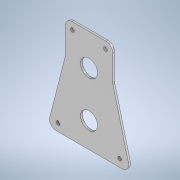
# Autodesk Inventor part: TH22_AlBoard_roller_sub_sn
Saved by Autodesk Inventor 2022 (Build 260153000, 153)
## iProperties
Created: 2022-02-09
Part Number: TH22_AlBoard_roller_sub_sn
Material: アルミニウム 6061-AHC
Document SubType Name: Modeling
Designer: 中島 青蔵
Density: 2.7 g/cm^3
Appearance: アルミニウム - ダーク
Author: 中島 青蔵
Autodesk Inventor part; units mm, degrees
ref_plane "YZ Plane" through (0, 0, 0) normal (1, 0, 0) x (0, 1, 0)
ref_plane "XZ Plane" through (0, 0, 0) normal (0, 1, 0) x (-1, 0, 0)
ref_plane "XY Plane" through (0, 0, 0) normal (0, 0, 1) x (1, 0, 0)
sketch "スケッチ1" plane through (0, 0, 0) normal (0, 0, 1) x (1, 0, 0)
  line L0 (0, 0) -> (50, 0)
  line L1 (50, 0) -> (50, 115)
  line L2 (50, 115) -> (0, 115)
  line L3 (0, 115) -> (0, 0)
  circle A0 centre (25, 81.5) radius 9
  circle A1 centre (25, 33.5) radius 9
  line L4 (0, 0) -> (-18.7939, 6.8404)
  line L5 (-18.7939, 6.8404) -> (0, 80)
  line L6 (50, 0) -> (68.7939, 6.8404)
  line L7 (68.7939, 6.8404) -> (50, 80)
  line L8 (-18.7939, 6.8404) -> (68.7939, 6.8404)
  dimension "d0" = 50
  dimension "d1" = 115
  dimension "d2" = 18
  dimension "d3" = 18
  dimension "d5" = 48
  dimension "d8" = 33.5
  dimension "d27" = 20
  dimension "d28" = 20
  dimension "d34" = 80
  dimension "d35" = 80
  dimension "d36" = 20
  dimension "d37" = 20
  constraints: 18 end point, 2 centre point, 2 parallel, 2 point on line, 1 horizontal, 1 vertical
  measures "d0" distance of L2.end L1.end
  measures "d1" distance of L1.end L0.end
  measures "d2" diameter of A0
  measures "d3" diameter of A1
  measures "d5" distance of A1.centre A0.centre
  measures "d8" distance from line of L0 A1.centre
  measures "d27" distance of L0.start L4.end
  measures "d28" distance of L6.end L0.end
  measures "d34" distance from line of L0 L5.end
  measures "d35" distance from line of L0 L7.end
  measures "d36" angle of L0 L6
  measures "d37" angle of L0 L4
extrude "押し出し1" add sketch "スケッチ1" along normal blind 2 contours L8 L5 L3 | L3 L2 L1 L8 | L1 L7 L8
sketch "スケッチ2" plane through (0, 0, 2) normal (0, 0, 1) x (1, 0, 0)
  line L0 (0, 115) -> (0, 0) projected
  line L1 (50, 80) -> (50, 115) projected
  line L2 (50, 115) -> (0, 115) projected
  point P0 (7.5, 107.5)
  point P1 (42.5, 107.5)
  point P2 (57.5, 15)
  point P3 (-7.5, 15)
  dimension "d15" = 7.5
  dimension "d16" = 7.5
  dimension "d17" = 7.5
  dimension "d18" = 7.5
  dimension "d31" = 7.5
  dimension "d32" = 7.5
  dimension "d40" = 15
  dimension "d41" = 15
  measures "d15" distance from line of L2 point (7.5, 107.5)
  measures "d16" distance from line of L0 point (7.5, 107.5)
  measures "d17" distance from line of L1 point (42.5, 107.5)
  measures "d18" distance from line of L2 point (42.5, 107.5)
  measures "d31" distance from line of L0 point (-7.5, 15)
  measures "d32" distance from line of L1 point (57.5, 15)
  measures "d40" vertical distance of L0.end point (57.5, 15)
  measures "d41" vertical distance of L0.end point (-7.5, 15)
hole "穴1" at (7.5, 107.5, 2) at (42.5, 107.5, 2) at (57.5, 15, 2) at (-7.5, 15, 2) direction (0, 0, -1) diameter 4 depth 8 tip angle 118
fillet "フィレット2" radius 7 6 edges at (50, 115, 1) (0, 115, 1) (0, 80, 1) (50, 80, 1) (-18.7939, 6.8404, 1) (68.7939, 6.8404, 1)
equation "\"d8\" = -0.5 * d5 + 0.5 * d1"
equation "\"d35\" = d34"
equation "\"d37\" = d36"
equation "\"d15\" = d18"
equation "\"d16\" = d18"
equation "\"d17\" = d18"
equation "\"d31\" = d18"
equation "\"d32\" = d18"
equation "\"d41\" = d40"
